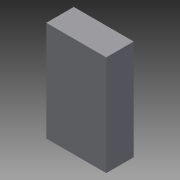
# Autodesk Inventor part: usb hub d link
Saved by Autodesk Inventor 2015 (Build 190159000, 159)
## iProperties
Created: 2014-09-17
Part Number: usb hub d link
Material: Generic
Document SubType Name: Modeling
Designer: ericd_000
Density: 1 g/cm^3
Appearance: Default
Author: ericd_000
Autodesk Inventor part; units mm, degrees
ref_plane "YZ Plane" through (0, 0, 0) normal (1, 0, 0) x (0, 1, 0)
ref_plane "XZ Plane" through (0, 0, 0) normal (0, 1, 0) x (-1, 0, 0)
ref_plane "XY Plane" through (0, 0, 0) normal (0, 0, 1) x (1, 0, 0)
sketch "Sketch1" plane through (0, 0, 0) normal (0, 1, 0) x (-1, 0, 0)
  line L0 (28.7306, 48.8204) -> (-32.2694, 48.8204)
  line L1 (-32.2694, 48.8204) -> (-32.2694, -53.1796)
  line L2 (-32.2694, -53.1796) -> (28.7306, -53.1796)
  line L3 (28.7306, -53.1796) -> (28.7306, 48.8204)
  point P0 (0, 0)
  dimension "d0" = 102
  dimension "d1" = 61
  constraints: 8 end point, 2 parallel, 1 horizontal, 1 perpendicular
  measures "d0" distance of L2.end L0.start
  measures "d1" distance of L0.start L0.end
extrude "Extrusion1" add sketch "Sketch1" along normal blind 28
body "Solid1"
